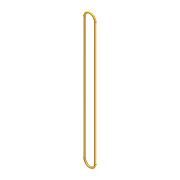
# Autodesk Inventor part: Belt_VerticalConveyor_Rear
Saved by Autodesk Inventor 2012 (Build 160160000, 160)
## iProperties
Created: 2012-01-21
Part Number: Belt_VerticalConveyor_Rear
Material: Default
Document SubType Name: Modeling
Designer: JesseK
Density: 1 g/cm^3
Mass: 21.727 g
Surface Area: 182.365 cm^2
Volume: 21.727 cm^3
Author: JesseK
Autodesk Inventor part; units mm, degrees
ref_plane "YZ Plane" through (0, 0, 0) normal (1, 0, 0) x (0, 1, 0)
ref_plane "XZ Plane" through (0, 0, 0) normal (0, 1, 0) x (-1, 0, 0)
ref_plane "XY Plane" through (0, 0, 0) normal (0, 0, 1) x (1, 0, 0)
sketch "Sketch1" plane through (0, 0, 0) normal (0, 0, 1) x (1, 0, 0)
  arc A0 (-19.05, 0) -> (19.05, 0) centre (0, 0) ccw
  arc A1 (19.05, 469.9) -> (-19.05, 469.9) centre (0, 469.9) ccw
  line L0 (-19.05, 0) -> (-19.05, 469.9)
  line L1 (19.05, 469.9) -> (19.05, 0)
  arc A2 (23.8125, 469.9) -> (-23.8125, 469.9) centre (0, 469.9) ccw
  arc A3 (-23.8125, 0) -> (23.8125, 0) centre (0, 0) ccw
  line L2 (-23.8125, 469.9) -> (-23.8125, 0)
  line L3 (23.8125, 0) -> (23.8125, 469.9)
  dimension "d0" = 469.9
  dimension "d1" = 19.05
  dimension "d2" = 4.7625
  constraints: 8 end point, 8 point on circle, 8 tangent, 4 centre point, 4 vertical, 3 coincident
  measures "d0" distance of L1.start L1.end
  measures "d1" radius of A0
  measures "d2" distance between parallel lines of L0 L2
extrude "Extrusion1" add sketch "Sketch1" along normal blind 4.7625
fillet "Fillet1" radius 2.3813 8 edges at (0, 493.7125, 4.7625) (23.8125, 234.95, 4.7625) (0, -23.8125, 4.7625) (-23.8125, 234.95, 4.7625) (0, -23.8125, 0) (23.8125, 234.95, 0) (0, 493.7125, 0) (-23.8125, 234.95, 0)
body "Solid1"
